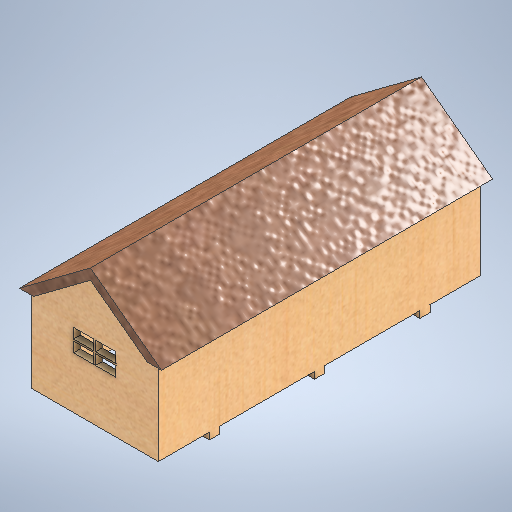
# Autodesk Inventor part: prvni navrh
Saved by Autodesk Inventor 2025.1 (Build 291241000, 241)
## iProperties
Created: 2024-10-27
Part Number: prvni navrh
Material: Všeobecné
Document SubType Name: Modeling
Designer: nelan
Density: 1 g/cm^3
Appearance: 1.5palcový čtverec – střední modrá
Author: nelan
Autodesk Inventor part; units mm, degrees
ref_plane "XZ Plane" through (0, 0, 0) normal (0, 1, 0) x (-1, 0, 0)
ref_plane "XY Plane" through (0, 0, 0) normal (0, 0, 1) x (1, 0, 0)
sketch "Náčrt1" plane through (0, 0, 0) normal (1, 0, 0) x (0, 1, 0)
  line L0 (25, 95) -> (-25, 95)
  line L1 (-25, 95) -> (-25, -95)
  line L2 (-25, -95) -> (25, -95)
  line L3 (25, -95) -> (25, 95)
  line L4 (25, 95) -> (-25, -95) construction
  line L5 (-25, 95) -> (25, -95) construction
  line L6 (-25, -3) -> (-29, -3)
  line L7 (-29, -3) -> (-29, 3)
  line L8 (-29, 3) -> (-25, 3)
  line L9 (-25, 3) -> (-25, -3)
  line L10 (-25, -65) -> (-29, -65)
  line L11 (-29, -65) -> (-29, -59)
  line L12 (-29, -59) -> (-25, -59)
  line L13 (-25, -59) -> (-25, -65)
  line L14 (-25, 59) -> (-29, 59)
  line L15 (-29, 59) -> (-29, 65)
  line L16 (-29, 65) -> (-25, 65)
  line L17 (-25, 65) -> (-25, 59)
  line L18 (7.5, 95) -> (7.5, 85)
  line L19 (7.5, 85) -> (17.5, 85)
  line L20 (17.5, 85) -> (17.5, 95)
  line L21 (-3.3333, 95) -> (-3.3333, 85)
  line L22 (-3.3333, 85) -> (-13.3333, 85)
  line L23 (-13.3333, 85) -> (-13.3333, 95)
  point P0 (0, 0)
  point P1 (25, 0)
  point P2 (-25, 0)
  point P3 (-25, 0)
  point P4 (-27, 3)
  point P5 (-27, 59)
  point P6 (12.5, 85)
  point P7 (-8.3333, 85)
  dimension "d0" = 50
  dimension "d1" = 190
  dimension "d46" = 6
  dimension "d47" = 4
  dimension "d48" = 4
  dimension "d49" = 6
  dimension "d50" = 30
  dimension "d51" = 4
  dimension "d52" = 6
  dimension "d53" = 30
  dimension "d54" = 56
  dimension "d73" = 10
  dimension "d74" = 10
  dimension "d75" = 10
  dimension "d76" = 10
  dimension "d77" = 12.5
  dimension "d78" = 16.6667
  constraints: 48 end point, 9 midpoint, 8 parallel, 8 perpendicular, 7 point on line, 4 horizontal, 2 vertical, 1 coincident
  measures "d0" distance of L2.end L1.end
  measures "d1" distance of L1.end L0.end
  measures "d46" distance of L6.end L7.end
  measures "d47" distance of L7.end L8.end
  measures "d48" distance of L11.end L12.end
  measures "d49" distance of L10.end L11.end
  measures "d50" distance from line of L10 L1.end
  measures "d51" distance of L15.end L16.end
  measures "d52" distance of L14.end L15.end
  measures "d53" distance from line of L0.end L16
  measures "d54" distance of point (-27, 3) point (-27, 59)
  measures "d73" distance of L21.end L22.end
  measures "d74" distance of L18.end L19.end
  measures "d75" distance between parallel lines of L0 L19
  measures "d76" distance between parallel lines of L0 L22
  measures "d77" distance from line of L3 point (12.5, 85)
  measures "d78" distance from line of L1 point (-8.333, 85)
extrude "Vysunutí1" add sketch "Náčrt1" against normal blind 4
sketch "Náčrt2" plane through (0, 0, 0) normal (0, 0, 1) x (1, 0, 0)
  line L0 (-4, -25) -> (-4, 25) projected
  line L1 (4.3597, 25) -> (-37.5, 56.2403)
  line L2 (4.3597, 25) -> (-4, 25)
  line L3 (-4, 25) -> (-37.5, 50.0013)
  line L4 (-37.5, 56.2403) -> (-37.5, 50.0013)
  line L5 (0, -25) -> (0, 25) projected
  point P0 (0, 0)
  dimension "d56" = 31.2403
  dimension "d57" = 33.5
  dimension "d65" = 5
  constraints: 8 end point, 1 coincident, 1 horizontal, 1 horizontal alignment, 1 parallel, 1 vertical
  measures "d56" vertical distance of L1.end L1.start
  measures "d57" horizontal distance of L2.end L1.end
  measures "d65" distance between parallel lines of L1 L3
extrude "Vysunutí3" add sketch "Náčrt2" along normal mid plane 195
ref_plane "Pracovní rovina2" through (-37.5, 0, 0) normal (1, 0, 0) x (0, 1, 0)
mirror "Zrcadlit2" about plane through (-37.5, 0, 0) normal (1, 0, 0) of "Vysunutí3", "Vysunutí1"
sketch "Náčrt4" plane through (-4, -25, 95) normal (0, 0, 1) x (1, 0, 0)
  line L0 (4, 0) -> (0, 0) projected
  line L1 (-67, 50) -> (0, 50)
  line L2 (0, 50) -> (0, 0)
  line L3 (0, 0) -> (-67, 0)
  line L4 (-67, 0) -> (-67, 50)
  line L5 (-46, 43.5) -> (-21, 43.5)
  line L6 (-21, 43.5) -> (-21, 30.5)
  line L7 (-21, 30.5) -> (-46, 30.5)
  line L8 (-46, 30.5) -> (-46, 43.5)
  line L9 (-46, 43.5) -> (-21, 30.5) construction
  line L10 (-21, 43.5) -> (-46, 30.5) construction
  line L11 (-33, 43.5) -> (-33, 30.5)
  line L12 (-34, 43.5) -> (-34, 30.5)
  line L13 (-46, 37.5) -> (-21, 37.5)
  line L14 (-46, 36.5) -> (-21, 36.5)
  point P0 (4, 25)
  point P1 (-33.5, 37)
  point P2 (-33.5, 50)
  point P3 (-34, 36.5)
  point P4 (-33, 36.5)
  point P5 (-33, 37.5)
  point P6 (-34, 37.5)
  dimension "d30" = 50
  dimension "d31" = 67
  dimension "d34" = 25
  dimension "d35" = 13
  dimension "d37" = 21
  dimension "d38" = 1
  dimension "d39" = 1
  dimension "d41" = 6
  dimension "d42" = 12
  dimension "d43" = 25
  dimension "d66" = 6.5
  constraints: 28 end point, 7 point on line, 6 perpendicular, 4 parallel, 3 midpoint, 2 horizontal
  measures "d30" distance between parallel lines of L3 L1
  measures "d31" distance between parallel lines of L2 L4
  measures "d34" distance of L6.end L7.end
  measures "d35" distance of L5.end L6.end
  measures "d37" distance between parallel lines of L2 L6
  measures "d38" distance between parallel lines of L11 L12
  measures "d39" distance between parallel lines of L14 L13
  measures "d41" distance between parallel lines of L5 L13
  measures "d42" distance between parallel lines of L6 L11
  measures "d43" distance of L13.start L13.end
  measures "d66" distance between parallel lines of L1 L5
extrude "Vysunutí5" add sketch "Náčrt4" against normal blind 4 contours L1 L2 L3 L4 | L5 L12 L13 L8 | L5 L11 L13 L12 | L13 L12 L14 L8 | L5 L6 L13 L11 | L13 L11 L14 L12 | L14 L12 L7 L8 | L13 L6 L14 L11 | L14 L11 L7 L12 | L14 L6 L7 L11
extrude "Vysunutí6" cut sketch "Náčrt4" against normal blind 10 contours L5 L12 L13 L8 | L5 L6 L13 L11 | L14 L12 L7 L8 | L14 L6 L7 L11
sketch "Náčrt5" plane through (0, -25, -95) normal (0, 0, -1) x (-1, 0, 0)
  line L0 (4, 50) -> (37.5, 75.0013) projected
  line L1 (4, 50) -> (71, 50)
  line L2 (4, 50) -> (37.5, 75.0013)
  line L3 (37.5, 75.0013) -> (71, 50) projected
  line L4 (37.5, 75.0013) -> (71, 50)
  line L5 (71, 50) -> (37.5, 75.0013) projected
  point P0 (0, 25)
  dimension "d67" = 67
  constraints: 6 end point, 2 point on line, 1 collinear
  measures "d67" distance of L0.start L1.end
extrude "Vysunutí7" add sketch "Náčrt5" against normal blind 4
mirror "Zrcadlit4" about plane through (0, 0, 0) normal (0, 0, 1) of "Vysunutí7"
